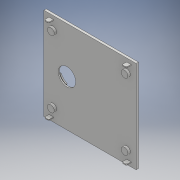
# Autodesk Inventor part: Top Roof
Saved by Autodesk Inventor 2017 (Build 210142000, 142)
## iProperties
Created: 2018-02-08
Part Number: Top Roof
Material: Generic
Document SubType Name: Modeling
Designer: Arjuna
Density: 1 g/cm^3
Appearance: Default
Author: Arjuna
Autodesk Inventor part; units mm, degrees
ref_plane "YZ Plane" through (0, 0, 0) normal (1, 0, 0) x (0, 1, 0)
ref_plane "XZ Plane" through (0, 0, 0) normal (0, 1, 0) x (-1, 0, 0)
ref_plane "XY Plane" through (0, 0, 0) normal (0, 0, 1) x (1, 0, 0)
sketch "Sketch1" plane through (0, 0, 0) normal (0, 1, 0) x (-1, 0, 0)
  line L0 (-100, 100) -> (100, 100)
  line L1 (100, 100) -> (100, -100)
  line L2 (100, -100) -> (-100, -100)
  line L3 (-100, -100) -> (-100, 100)
  point P0 (0, 0)
  dimension "d0" = 200
  dimension "d1" = 200
  dimension "d2" = 100
  dimension "d3" = 100
  constraints: 8 end point, 2 parallel, 1 horizontal, 1 perpendicular
  measures "d0" distance between parallel lines of L2 L0
  measures "d1" distance between parallel lines of L3 L1
  measures "d2" distance from line of point (0, 0) L1
  measures "d3" distance from line of point (0, 0) L0
extrude "Extrusion1" add sketch "Sketch1" along normal blind 5
sketch "Sketch2" plane through (0, 5, 0) normal (0, 1, 0) x (1, 0, 0)
  circle A0 centre (-50, 0) radius 19
  point P0 (0, 0)
  dimension "d6" = 38
  dimension "d7" = 50
  constraints: 1 centre point
  measures "d6" diameter of A0
  measures "d7" distance of point (0, 0) A0.centre
extrude "Extrusion2" cut sketch "Sketch2" against normal through all
sketch "Sketch3" plane through (0, 0, 0) normal (0, -1, 0) x (1, 0, 0)
  circle A0 centre (-80, -72.5) radius 7.5
  circle A1 centre (-80, 72.5) radius 7.5
  circle A2 centre (80, -72.5) radius 7.5
  circle A3 centre (80, 72.5) radius 7.5
  circle A4 centre (-80, -72.5) radius 8.5
  circle A5 centre (-80, 72.5) radius 8.5
  circle A6 centre (80, 72.5) radius 8.5
  circle A7 centre (80, -72.5) radius 8.5
  point P0 (0, 0)
  dimension "d10" = 15
  dimension "d11" = 72.5
  dimension "d12" = 80
  dimension "d13" = 15
  dimension "d14" = 72.5
  dimension "d15" = 80
  dimension "d16" = 15
  dimension "d17" = 15
  dimension "d18" = 72.5
  dimension "d19" = 72.5
  dimension "d20" = 80
  dimension "d21" = 80
  dimension "d22" = 17
  dimension "d23" = 17
  dimension "d24" = 17
  dimension "d25" = 17
  constraints: 8 centre point, 4 coincident
  measures "d10" diameter of A0
  measures "d11" vertical distance of point (0, 0) A0.centre
  measures "d12" horizontal distance of point (0, 0) A0.centre
  measures "d13" diameter of A1
  measures "d14" vertical distance of point (0, 0) A1.centre
  measures "d15" horizontal distance of point (0, 0) A1.centre
  measures "d16" diameter of A2
  measures "d17" diameter of A3
  measures "d18" vertical distance of point (0, 0) A2.centre
  measures "d19" vertical distance of point (0, 0) A3.centre
  measures "d20" horizontal distance of point (0, 0) A3.centre
  measures "d21" horizontal distance of point (0, 0) A2.centre
  measures "d22" diameter of A4
  measures "d23" diameter of A5
  measures "d24" diameter of A7
  measures "d25" diameter of A6
extrude "Extrusion3" [suppressed]
sketch "Sketch4" plane through (0, 5, 0) normal (0, 1, 0) x (1, 0, 0)
  circle A0 centre (-50, 0) radius 19
  circle A1 centre (-50, 0) radius 22
  point P0 (0, 0)
  dimension "d28" = 44
  constraints: 2 centre point, 1 coincident
  measures "d28" diameter of A1
extrude "Extrusion4" cut sketch "Sketch4" against normal blind 2.5
extrude "Extrusion5" add sketch "Sketch3" along normal blind 5 contours A0 | A1 | A2 | A3
sketch "Sketch5" plane through (0, 0, 0) normal (0, -1, 0) x (1, 0, 0)
  line L0 (-115, -92.5) -> (-115, 92.5)
  line L1 (-115, -92.5) -> (115, -92.5)
  line L2 (-115, 92.5) -> (115, 92.5)
  line L3 (115, 92.5) -> (115, -92.5)
  line L4 (-89, -92.5) -> (-79.5, -92.5)
  line L5 (-79.5, -92.5) -> (-79.5, -90.5)
  line L6 (-79.5, -90.5) -> (-89, -90.5)
  line L7 (-89, -90.5) -> (-89, -92.5)
  line L8 (-89, 92.5) -> (-79.5, 92.5)
  line L9 (-79.5, 92.5) -> (-79.5, 90.5)
  line L10 (-79.5, 90.5) -> (-89, 90.5)
  line L11 (-89, 90.5) -> (-89, 92.5)
  line L12 (79.5, -92.5) -> (89, -92.5)
  line L13 (89, -92.5) -> (89, -90.5)
  line L14 (89, -90.5) -> (79.5, -90.5)
  line L15 (79.5, -90.5) -> (79.5, -92.5)
  line L16 (79.5, 92.5) -> (89, 92.5)
  line L17 (89, 92.5) -> (89, 90.5)
  line L18 (89, 90.5) -> (79.5, 90.5)
  line L19 (79.5, 90.5) -> (79.5, 92.5)
  point P0 (0, 0)
  dimension "d33" = 185
  dimension "d34" = 92.5
  dimension "d35" = 230
  dimension "d36" = 115
  dimension "d37" = 9.5
  dimension "d38" = 2
  dimension "d39" = 26
  dimension "d40" = 9.5
  dimension "d41" = 2
  dimension "d42" = 26
  dimension "d43" = 9.5
  dimension "d44" = 2
  dimension "d45" = 26
  dimension "d46" = 2
  dimension "d47" = 9.5
  dimension "d48" = 26
  dimension "d90" = 159
  constraints: 40 end point, 8 parallel, 6 horizontal, 5 perpendicular, 4 point on line, 1 vertical
  measures "d33" distance of L0.start L0.end
  measures "d34" vertical distance of point (0, 0) L0.start
  measures "d35" distance of L0.start L1.end
  measures "d36" horizontal distance of point (0, 0) L0.start
  measures "d37" distance of L6.end L5.end
  measures "d38" distance between parallel lines of L6 L1
  measures "d39" distance between parallel lines of L7 L0
  measures "d40" distance between parallel lines of L9 L11
  measures "d41" distance between parallel lines of L8 L10
  measures "d42" distance between parallel lines of L11 L0
  measures "d43" distance of L14.end L13.end
  measures "d44" distance between parallel lines of L14 L1
  measures "d45" distance between parallel lines of L3 L13
  measures "d46" distance between parallel lines of L16 L18
  measures "d47" distance between parallel lines of L17 L19
  measures "d48" distance between parallel lines of L3 L17
  measures "d90" distance of L16.start L8.end
extrude "Extrusion6" add sketch "Sketch5" along normal blind 10 contours L7 L6 L5 L1 | L2 L9 L10 L11 | L15 L14 L13 L1 | L2 L17 L18 L19
chamfer "Chamfer1" distance 2 angle 45 8 edges at (-79.5, -10, -91.5) (-89, -10, -91.5) (-79.5, -10, 91.5) (-89, -10, 91.5) (79.5, -10, 91.5) (89, -10, 91.5) (89, -10, -91.5) (79.5, -10, -91.5)
sketch "Sketch6" plane through (0, 5, 0) normal (0, 1, 0) x (1, 0, 0)
  circle A0 centre (-50, 0) radius 19
  circle A1 centre (-50, 0) radius 22
  circle A2 centre (-50, 0) radius 29.5
  circle A3 centre (-50, 0) radius 32.5
  point P0 (0, 0)
  dimension "d54" = 59
  dimension "d57" = 65
  dimension "d58" = 3
  constraints: 4 centre point, 1 coincident
  measures "d54" diameter of A2
  measures "d57" diameter of A3
  measures "d58" radial gap between concentric circles of A3 A2
extrude "Extrusion7" add sketch "Sketch6" along normal blind 5 contours A3
sketch "Sketch7" plane through (-50, 10, 0) normal (0, 1, 0) x (-1, 0, 0)
  circle A0 centre (0, 0) radius 29.5 projected
  circle A1 centre (0, 0) radius 32.5 projected
  circle A2 centre (0, 0) radius 24.5
  point P0 (-50, 0)
  dimension "d61" = 49
  dimension "d62" = 5
  constraints: 1 centre point, 1 coincident
  measures "d61" diameter of A2
  measures "d62" radial gap between concentric circles of A0 A2
extrude "Extrusion8" add sketch "Sketch7" against normal blind 2.5 contours A0
sketch "Sketch8" plane through (-50, 10, 0) normal (0, 1, 0) x (1, 0, 0)
  circle A0 centre (0, 0) radius 24.5
  circle A1 centre (0, 0) radius 32.5
  line L0 (0, 0) -> (-32.5, 0)
  arc A2 (-30.0261, 12.4372) -> (-32.5, 0) centre (0, 0) ccw
  line L1 (0, 0) -> (-30.0261, 12.4372) construction
  line L2 (0, 0) -> (-32.5, 0) construction
  arc A3 (-32.5, 0) -> (-30.0261, -12.4372) centre (0, 0) ccw
  line L3 (0, 0) -> (-30.0261, -12.4372) construction
  line L4 (0, 0) -> (-32.5, 0) construction
  arc A4 (-22.635, 9.3757) -> (-24.5, 0) centre (0, 0) ccw
  line L5 (0, 0) -> (-22.635, 9.3757) construction
  line L6 (0, 0) -> (-24.5, 0) construction
  arc A5 (-24.5, 0) -> (-22.635, -9.3757) centre (0, 0) ccw
  line L7 (0, 0) -> (-22.635, -9.3757) construction
  line L8 (0, 0) -> (-24.5, 0) construction
  line L9 (-30.0261, -12.4372) -> (-22.635, -9.3757)
  line L10 (-30.0261, 12.4372) -> (-22.635, 9.3757)
  line L11 (-12.4372, -30.0261) -> (-9.3757, -22.635)
  arc A6 (-12.4372, -30.0261) -> (0, -32.5) centre (0, 0) ccw
  arc A7 (0, -24.5) -> (9.3757, -22.635) centre (0, 0) ccw
  line L12 (12.4372, -30.0261) -> (9.3757, -22.635)
  arc A8 (0, -32.5) -> (12.4372, -30.0261) centre (0, 0) ccw
  arc A9 (-9.3757, -22.635) -> (0, -24.5) centre (0, 0) ccw
  line L13 (30.0261, -12.4372) -> (22.635, -9.3757)
  arc A10 (30.0261, -12.4372) -> (32.5, 0) centre (0, 0) ccw
  arc A11 (24.5, 0) -> (22.635, 9.3757) centre (0, 0) ccw
  line L14 (30.0261, 12.4372) -> (22.635, 9.3757)
  arc A12 (32.5, 0) -> (30.0261, 12.4372) centre (0, 0) ccw
  arc A13 (22.635, -9.3757) -> (24.5, 0) centre (0, 0) ccw
  line L15 (12.4372, 30.0261) -> (9.3757, 22.635)
  arc A14 (12.4372, 30.0261) -> (0, 32.5) centre (0, 0) ccw
  arc A15 (0, 24.5) -> (-9.3757, 22.635) centre (0, 0) ccw
  line L16 (-12.4372, 30.0261) -> (-9.3757, 22.635)
  arc A16 (0, 32.5) -> (-12.4372, 30.0261) centre (0, 0) ccw
  arc A17 (9.3757, 22.635) -> (0, 24.5) centre (0, 0) ccw
  point P0 (-50, 0)
  dimension "d65" = 22.5
  dimension "d66" = 22.5
  dimension "d67" = 22.5
  dimension "d68" = 22.5
  dimension "d71" = 360
  constraints: 34 end point, 32 point on circle, 16 centre point, 13 coincident, 2 horizontal alignment, 1 horizontal, 1 point on line, 69 other
  measures "d65" angle of L1 L2
  measures "d66" angle of L4 L3
  measures "d67" angle of L5 L6
  measures "d68" angle of L8 L7
extrude "Extrusion9" cut sketch "Sketch8" against normal up to surface (5 mm away) contours A0 L14 A1 L13 | A0 L16 A1 L15 | L12 A1 L11 A0 | A0 L0 A1 L10 | L9 A1 L0 A0
sketch "Sketch9" plane through (-50, 7.5, 0) normal (0, -1, 0) x (-1, 0, 0)
  arc A0 (22.635, 9.3757) -> (9.3757, 22.635) centre (0, 0) ccw projected
  line L0 (11.2892, 27.2544) -> (9.3757, 22.635) projected
  arc A1 (30.0261, 12.4372) -> (12.4372, 30.0261) centre (0, 0) ccw projected
  arc A2 (22.635, 9.3757) -> (9.3757, 22.635) centre (0, 0) ccw projected
  line L1 (-9.3754, -22.6343) -> (-12.4372, -30.0261)
  line L2 (-9.3754, -22.6343) -> (-12.4372, -30.0261)
  line L3 (-12.2788, -21.4249) -> (-15.2846, -28.6816)
  line L4 (-12.2788, -21.4249) -> (-12.2036, -21.2434)
  arc A3 (-12.2036, -21.2434) -> (-9.3754, -22.6343) centre (0, 0) ccw
  arc A4 (-15.2846, -28.6816) -> (-12.4372, -30.0261) centre (0, 0) ccw
  arc A5 (-22.635, -9.3757) -> (-9.3757, -22.635) centre (0, 0) ccw projected
  arc A6 (-30.0261, -12.4372) -> (-12.4372, -30.0261) centre (0, 0) ccw projected
  arc A7 (-12.4372, 30.0261) -> (-30.0261, 12.4372) centre (0, 0) ccw projected
  arc A8 (-9.3757, 22.635) -> (-22.635, 9.3757) centre (0, 0) ccw projected
  arc A9 (9.3757, -22.635) -> (22.635, -9.3757) centre (0, 0) ccw projected
  arc A10 (12.4372, -30.0261) -> (30.0261, -12.4372) centre (0, 0) ccw projected
  line L5 (21.4249, -12.2788) -> (21.2434, -12.2036)
  arc A11 (21.2434, -12.2036) -> (22.6343, -9.3754) centre (0, 0) ccw
  line L6 (21.4249, -12.2788) -> (28.6816, -15.2846)
  line L7 (22.6343, -9.3754) -> (30.0261, -12.4372)
  line L8 (22.6343, -9.3754) -> (30.0261, -12.4372)
  arc A12 (28.6816, -15.2846) -> (30.0261, -12.4372) centre (0, 0) ccw
  line L9 (12.2788, 21.4249) -> (12.2036, 21.2434)
  arc A13 (12.2036, 21.2434) -> (9.3754, 22.6343) centre (0, 0) ccw
  line L10 (12.2788, 21.4249) -> (15.2846, 28.6816)
  line L11 (9.3754, 22.6343) -> (12.4372, 30.0261)
  line L12 (9.3754, 22.6343) -> (12.4372, 30.0261)
  arc A14 (15.2846, 28.6816) -> (12.4372, 30.0261) centre (0, 0) ccw
  line L13 (-21.4249, 12.2788) -> (-21.2434, 12.2036)
  arc A15 (-21.2434, 12.2036) -> (-22.6343, 9.3754) centre (0, 0) ccw
  line L14 (-21.4249, 12.2788) -> (-28.6816, 15.2846)
  line L15 (-22.6343, 9.3754) -> (-30.0261, 12.4372)
  line L16 (-22.6343, 9.3754) -> (-30.0261, 12.4372)
  arc A16 (-28.6816, 15.2846) -> (-30.0261, 12.4372) centre (0, 0) ccw
  line L17 (12.4372, -30.0261) -> (9.3757, -22.635) projected
  line L18 (22.635, -9.3757) -> (30.0261, -12.4372) projected
  line L19 (-22.635, 9.3757) -> (-30.0261, 12.4372) projected
  line L20 (-12.4372, 30.0261) -> (-9.3757, 22.635) projected
  line L21 (-30.0261, -12.4372) -> (-22.635, -9.3757) projected
  line L22 (-9.3757, -22.635) -> (-12.4372, -30.0261) projected
  line L23 (9.3757, 22.635) -> (12.4372, 30.0261) projected
  line L24 (30.0261, 12.4372) -> (22.635, 9.3757) projected
  point P0 (-50, 0)
  dimension "d80" = 360
  constraints: 32 end point, 17 point on circle, 8 centre point, 5 coincident, 1 collinear, 53 other
extrude "Extrusion10" add sketch "Sketch9" along normal up to surface (7.5 mm away) contours A0 L0 L11 A1 L10 L9 | L1 A4 L3 L4 A3 | L14 L13 A8 L15 A7 | A9 L7 A10 L6 L5
sketch "Sketch10" plane through (-50, 7.5, 0) normal (0, -1, 0) x (-1, 0, 0)
  arc A0 (9.3757, -22.635) -> (22.635, -9.3757) centre (0, 0) ccw projected
  arc A1 (12.4372, -30.0261) -> (30.0261, -12.4372) centre (0, 0) ccw projected
  arc A2 (30.0261, 12.4372) -> (12.4372, 30.0261) centre (0, 0) ccw projected
  arc A3 (22.635, 9.3757) -> (9.3757, 22.635) centre (0, 0) ccw projected
  arc A4 (-12.4372, 30.0261) -> (-30.0261, 12.4372) centre (0, 0) ccw projected
  arc A5 (-9.3757, 22.635) -> (-22.635, 9.3757) centre (0, 0) ccw projected
  arc A6 (-22.635, -9.3757) -> (-9.3757, -22.635) centre (0, 0) ccw projected
  arc A7 (-30.0261, -12.4372) -> (-12.4372, -30.0261) centre (0, 0) ccw projected
  line L0 (-11.2892, -27.2544) -> (-9.3757, -22.635)
  arc A8 (-12.2421, -21.2222) -> (-9.3757, -22.635) centre (0, 0) ccw
  arc A9 (27.2544, 11.2892) -> (11.2892, 27.2544) centre (0, 0) ccw projected
  line L1 (-12.2421, -21.2222) -> (0, 0)
  arc A10 (-14.7405, -25.5532) -> (11.2892, 27.2544) centre (0, 0) ccw
  line L2 (-12.2421, -21.2222) -> (-14.7405, -25.5532)
  line L3 (21.2222, -12.2421) -> (25.5532, -14.7405)
  arc A11 (25.5532, -14.7405) -> (-27.2544, 11.2892) centre (0, 0) ccw
  arc A12 (21.2222, -12.2421) -> (22.635, -9.3757) centre (0, 0) ccw
  line L4 (27.2544, -11.2892) -> (22.635, -9.3757)
  line L5 (12.2421, 21.2222) -> (14.7405, 25.5532)
  arc A13 (14.7405, 25.5532) -> (-11.2892, -27.2544) centre (0, 0) ccw
  arc A14 (12.2421, 21.2222) -> (9.3757, 22.635) centre (0, 0) ccw
  line L6 (11.2892, 27.2544) -> (9.3757, 22.635)
  line L7 (-21.2222, 12.2421) -> (-25.5532, 14.7405)
  arc A15 (-25.5532, 14.7405) -> (27.2544, -11.2892) centre (0, 0) ccw
  arc A16 (-21.2222, 12.2421) -> (-22.635, 9.3757) centre (0, 0) ccw
  line L8 (-27.2544, 11.2892) -> (-22.635, 9.3757)
  line L9 (-30.0261, -12.4372) -> (-22.635, -9.3757) projected
  line L10 (-9.3757, -22.635) -> (-12.4372, -30.0261) projected
  line L11 (-22.635, 9.3757) -> (-30.0261, 12.4372) projected
  line L12 (-12.4372, 30.0261) -> (-9.3757, 22.635) projected
  line L13 (9.3757, 22.635) -> (12.4372, 30.0261) projected
  line L14 (30.0261, 12.4372) -> (22.635, 9.3757) projected
  line L15 (12.4372, -30.0261) -> (9.3757, -22.635) projected
  line L16 (22.635, -9.3757) -> (30.0261, -12.4372) projected
  point P0 (-50, 0)
  dimension "d86" = 360
  constraints: 21 point on circle, 18 end point, 8 centre point, 1 coincident, 1 point on line, 45 other
extrude "Extrusion11" add sketch "Sketch10" along normal up to surface (7.5 mm away) contours A0 L4 A10 L3 | A10 L2 A6 L0 | L5 A3 L6 A9 | A11 L7 A5 L8
equation "\"d2\" = 0.5 * d1"
equation "\"d3\" = 0.5 * d0"
equation "\"d13\" = d10"
equation "\"d14\" = d11"
equation "\"d15\" = d12"
equation "\"d16\" = d10"
equation "\"d17\" = d10"
equation "\"d18\" = d11"
equation "\"d19\" = d11"
equation "\"d20\" = d12"
equation "\"d21\" = d12"
equation "\"d23\" = d22"
equation "\"d24\" = d22"
equation "\"d25\" = d22"
equation "\"d34\" = 0.5 * d33"
equation "\"d36\" = 0.5 * d35"
equation "\"d40\" = d37"
equation "\"d41\" = d38"
equation "\"d42\" = d39"
equation "\"d43\" = d37"
equation "\"d44\" = d38"
equation "\"d45\" = d39"
equation "\"d46\" = d38"
equation "\"d47\" = d37"
equation "\"d48\" = d39"
body "Solid1"
